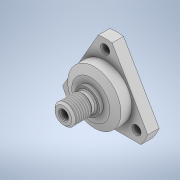
# Autodesk Inventor part: Люляев
Saved by Autodesk Inventor 2020 (Build 240168000, 168)
## iProperties
Created: 2020-05-25
Part Number: Люляев
Material: Типовые
Document SubType Name: Modeling
Designer: Сергей Ильин
Density: 1 g/cm^3
Appearance: По умолчанию
Author: Сергей Ильин
Autodesk Inventor part; units mm, degrees
ref_plane "YZ Plane" through (0, 0, 0) normal (1, 0, 0) x (0, 1, 0)
ref_plane "XZ Plane" through (0, 0, 0) normal (0, 1, 0) x (-1, 0, 0)
ref_plane "XY Plane" through (0, 0, 0) normal (0, 0, 1) x (1, 0, 0)
sketch "Эскиз1" plane through (0, 0, 0) normal (0, 0, 1) x (1, 0, 0)
  line L0 (9.0572, 59.3125) -> (55.8947, -21.8125)
  line L1 (46.8375, -37.5) -> (-46.8375, -37.5)
  line L2 (-55.8947, -21.8125) -> (-9.0572, 59.3125)
  arc A0 (9.0572, 59.3125) -> (-9.0572, 59.3125) centre (0, 0) ccw
  arc A1 (-55.8947, -21.8125) -> (-46.8375, -37.5) centre (0, 0) ccw
  arc A2 (46.8375, -37.5) -> (55.8947, -21.8125) centre (0, 0) ccw
  circle A3 centre (0, 47.5) radius 6
  circle A4 centre (-41.1362, -23.75) radius 6
  circle A5 centre (41.1362, -23.75) radius 6
  dimension "d3" = 12
  dimension "d6" = 360
  constraints: 6 centre point, 6 end point, 6 point on circle, 1 coincident, 11 other
  measures "d3" diameter of A3
extrude "Выдавливание1" add sketch "Эскиз1" along normal blind 15
sketch "Эскиз2" plane through (0, 0, 15) normal (0, 0, 1) x (1, 0, 0)
  circle A0 centre (0, 0) radius 35
  dimension "d10" = 70
  constraints: 1 centre point, 1 coincident
  measures "d10" diameter of A0
extrude "Выдавливание2" add sketch "Эскиз2" along normal blind 19
sketch "Эскиз3" plane through (0, 0, 0) normal (1, 0, 0) x (0, 1, 0)
  line L0 (-35, 15) -> (-35, 34) projected
  line L1 (35, 34) -> (-35, 34) projected
  line L2 (35, 15) -> (35, 34) projected
  line L3 (35, 29.3369) -> (25, 34)
  line L4 (0, 34) -> (0, 40.7436)
  point P0 (0, 0)
  dimension "d13" = 25
  dimension "d14" = 25
  constraints: 4 end point, 2 point on line, 2 vertical, 1 midpoint
  measures "d13" distance from line of L3.end L4
  measures "d14" angle of L1 L3
revolve "Вращение1" cut sketch "Эскиз3" angle 360 about axis through (0, 0, 34) along (0, 0, 1)
sketch "Эскиз4" plane through (0, 0, 34) normal (0, 0, 1) x (1, 0, 0)
  circle A0 centre (0, 0) radius 16.5
  dimension "d16" = 33
  constraints: 1 centre point, 1 coincident
  measures "d16" diameter of A0
extrude "Выдавливание3" add sketch "Эскиз4" along normal blind 5
sketch "Эскиз5" plane through (0, 0, 39) normal (0, 0, 1) x (1, 0, 0)
  circle A0 centre (0, 0) radius 13.5
  dimension "d19" = 27
  constraints: 1 centre point, 1 coincident
  measures "d19" diameter of A0
extrude "Выдавливание4" add sketch "Эскиз5" along normal blind 31
sketch "Эскиз6" plane through (0, 0, 0) normal (1, 0, 0) x (0, 1, 0)
  line L0 (-13.5, 39) -> (13.5, 39) projected
  line L1 (16.5, 39) -> (-16.5, 39) projected
  line L2 (13.5, 70) -> (-13.5, 70) projected
  line L3 (0, 70) -> (0, 78.8813)
  line L4 (12.1787, 39) -> (12.1787, 45)
  line L5 (12.1787, 45) -> (13.5, 46.3213)
  line L6 (13.5, 39) -> (13.5, 70) projected
  point P0 (0, 0)
  dimension "d22" = 45
  dimension "d23" = 6
  constraints: 6 end point, 2 point on line, 1 midpoint, 1 perpendicular, 1 vertical
  measures "d22" angle of L6 L5
  measures "d23" distance of L4.start L4.end
revolve "Вращение2" cut sketch "Эскиз6" angle 360 about axis through (0, 0, 70) along (0, 0, 1)
fillet "Сопряжение1" radius 1.6 1 edges at (0, -12.1787, 39)
fillet "Сопряжение2" radius 1 1 edges at (0, -12.1787, 45)
thread "Резьба1" size "M27x3" class "6g" standard "ISO Metric profile" full length
chamfer "Фаска1" distance 2.5 angle 45 1 edges at (-13.5, 0, 70)
sketch "Эскиз7" plane through (0, 0, 0) normal (0, 0, -1) x (-1, 0, 0)
  point P0 (0, 0)
  point P1 (0, 0)
  constraints: 1 coincident
hole "Отверстие1" at (0, 0, 0) direction (0, 0, 1) diameter 54 depth 10
sketch "Эскиз8" plane through (0, 0, 10) normal (0, 0, -1) x (-1, 0, 0)
  point P0 (0, 0)
  point P1 (0, 0)
  constraints: 1 coincident
sketch "Эскиз9" plane through (0, 0, 70) normal (0, 0, 1) x (1, 0, 0)
  point P0 (0, 0)
  point P1 (0, 0)
  constraints: 1 coincident
hole "Отверстие2" at (0, 0, 70) direction (0, 0, -1) diameter 12 depth 39
chamfer "Фаска2" distance 1 angle 45 1 edges at (0, 6, 70)
sketch "Эскиз10" plane through (0, 0, 31) normal (0, 0, 1) x (1, 0, 0)
  point P0 (0, 0)
  point P1 (0, 0)
  constraints: 1 coincident
hole "Отверстие3" at (0, 0, 31) direction (0, 0, -1) diameter 28 end through all
sketch "Эскиз11" plane through (0, 0, 0) normal (1, 0, 0) x (0, 1, 0)
  line L0 (14, 10) -> (-14, 10) projected
  line L1 (-27, 10) -> (27, 10) projected
  line L2 (-14, 31) -> (14, 31) projected
  line L3 (0, 10) -> (0, -15.8706)
  line L4 (20, 10) -> (14, 16)
  line L5 (14, 10) -> (-14, 10) projected
  line L6 (-14, 31) -> (14, 31) projected
  line L7 (14, 10) -> (14, 22.3316)
  line L8 (14, 10) -> (14, 31) projected
  point P0 (0, 0)
  dimension "d56" = 45
  dimension "d57" = 6
  constraints: 6 end point, 3 point on line, 1 midpoint, 1 vertical
  measures "d56" angle of L1 L4
  measures "d57" distance of L4.start L0.start
revolve "Вращение3" cut sketch "Эскиз11" angle 360 about axis through (0, 0, 10) along (0, 0, -1)
